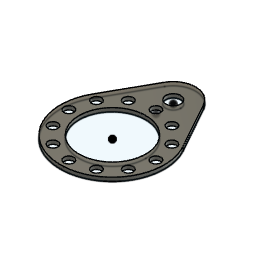
rod attachment v1 (Autodesk Fusion 360 design; units mm, degrees)
Autodesk Fusion 360 part; units mm, degrees
note: some values were not read from the file. Set by a fixed rule: the direction of a hole.
sketch "Sketch1" plane through (0, 0, 0) normal (0, 1, 0) x (1, 0, 0)
  circle A0 centre (0, 0) radius 22.5
  line L0 (-30.5533, 17.0732) -> (-13.0943, 48.3171)
  arc A1 (13.0943, 48.3171) -> (-13.0943, 48.3171) centre (0, 41) ccw
  line L1 (13.0943, 48.3171) -> (30.5533, 17.0732)
  arc A2 (-30.5533, 17.0732) -> (30.5533, 17.0732) centre (0, 0) ccw
  circle A3 centre (0, 41) radius 5
  point P0 (0, 29.35)
  dimension "d1" = 45
  dimension "d2" = 41
  dimension "d3" = 10
  dimension "d4" = 35
  dimension "d5" = 15
  dimension "d8" = 29.35
  constraint coincident A0.centre A2.centre
  constraint tangent L0 A1
  constraint tangent A1 L1
  constraint tangent L1 A2
  constraint tangent L0 A2
  constraint vertical A0.centre A1.centre
  constraint concentric A1 A3
  constraint vertical A0.centre P0
  measures "d1" diameter of A0
  measures "d2" distance of A0.centre A1.centre
  measures "d3" diameter of A3
  measures "d4" radius of A2
  measures "d5" radius of A1
  measures "d8" distance of A0.centre P0
extrude "Extrude1" add sketch "Sketch1" along normal blind 2.5
hole "Hole1" at (0, 0, -29.35) direction (0, 1, 0) diameter 6.6 end through all
pattern_circular "C-Pattern1" count 12 over 360 about axis through (0, 1.75, 0) along (0, 1, 0) of "Hole1"
equation "d8 = ( 58.7 / 2 ) * 1 mm"
